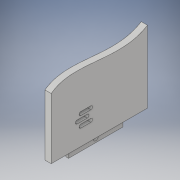
# Autodesk Inventor part: Case Left
Saved by Autodesk Inventor 2019 (Build 230136000, 136)
## iProperties
Created: 2022-04-25
Part Number: Case Left
Material: Generic
Document SubType Name: Modeling
Designer: Loxei
Density: 1 g/cm^3
Appearance: Default
Author: Loxei
Autodesk Inventor part; units mm, degrees
ref_plane "YZ Plane" through (0, 0, 0) normal (1, 0, 0) x (0, 1, 0)
ref_plane "XZ Plane" through (0, 0, 0) normal (0, 1, 0) x (-1, 0, 0)
ref_plane "XY Plane" through (0, 0, 0) normal (0, 0, 1) x (1, 0, 0)
sketch "Sketch2" plane through (0, 0, 0) normal (1, 0, 0) x (0, 1, 0)
  line L0 (43.74, 0) -> (-43.74, 0) construction
  line L1 (0, 65.172) -> (0, -65.172) construction
  spline S0 degree 3 poles (-5.8666, 35) (13.8832, 21.2522) (-10.0462, -16.0043) (8.551, -35) knots 1 1 1 1 2 2 2 2
  line L2 (-5.8666, 35) -> (13.8832, 21.2522) construction
  line L3 (13.8832, 21.2522) -> (-10.0462, -16.0043) construction
  line L4 (-10.0462, -16.0043) -> (8.551, -35) construction
  line L5 (-5.8666, 35) -> (-40.8666, 35)
  line L6 (-40.8666, 35) -> (-40.8666, 31)
  line L7 (-40.8666, 31) -> (-1.7165, 31)
  line L8 (-40.8666, 31) -> (-40.8666, -35)
  line L9 (-40.8666, -35) -> (8.551, -35)
  line L10 (-40.8666, -31) -> (5.392, -31)
  point P0 (0, 0)
  point P1 (0, 0)
  point P2 (0, 0)
  point P3 (0, 0)
  point P4 (-1.7165, 31)
  dimension "d0" = 35
  dimension "d1" = 4
  dimension "d2" = 4
  constraints: 16 end point, 4 midpoint, 3 perpendicular, 3 vertical, 2 horizontal, 2 parallel, 2 symmetric about line, 1 point on line, 6 other
  measures "d0" distance of L2.start L5.end
  measures "d1" distance of L5.end L6.end
  measures "d2" distance of L8.end L10.start
extrude "Extrusion1" add sketch "Sketch2" along normal blind 4 contours S0 L10 L8 L7
sketch "Sketch3" plane through (0, -40.8666, -31) normal (0, -1, 0) x (1, 0, 0)
  line L0 (0, 62) -> (0, 0) projected
  line L1 (0, 48.5) -> (1.7, 48.5)
  line L2 (1.7, 48.5) -> (1.7, 13.5)
  line L3 (1.7, 13.5) -> (0, 13.5)
  line L4 (0, 13.5) -> (0, 48.5)
  line L5 (0, 62) -> (4, 62) projected
  line L6 (0, 0) -> (4, 0) projected
  point P0 (0, 31)
  dimension "d5" = 1.7
  dimension "d6" = 35
  dimension "d7" = 13.5
  dimension "d8" = 13.5
  constraints: 8 end point, 2 parallel, 1 horizontal, 1 perpendicular, 1 point on line
  measures "d5" distance of L2.end L3.end
  measures "d6" distance of L1.end L2.end
  measures "d7" distance from line of L5 L1.start
  measures "d8" distance between parallel lines of L6 L3
extrude "Extrusion2" add sketch "Sketch3" along normal blind 4.9
chamfer "Chamfer1" distance 1.5 angle 45 1 edges at (1.7, -40.8666, 0)
sketch "Sketch4" plane through (0, 0, 0) normal (-1, 0, 0) x (0, 0, 1)
  circle A0 centre (22.15, -13.9166) radius 1.15
  circle A1 centre (22.15, -37.9166) radius 1.15
  line L0 (22.15, -13.9166) -> (22.15, -37.9166) construction
  circle A2 centre (-28.65, -13.9166) radius 1.15
  circle A3 centre (-28.65, -37.9166) radius 1.15
  line L1 (-28.65, -13.9166) -> (-28.65, -37.9166) construction
  line L2 (-28.65, -25.9166) -> (22.15, -25.9166) construction
  line L3 (-31, -40.8666) -> (-31, 5.392) projected
  line L4 (-17.5, -40.8666) -> (-31, -40.8666) projected
  point P0 (0, 0)
  dimension "d14" = 2.3
  dimension "d15" = 2.3
  dimension "d16" = 24
  dimension "d17" = 2.3
  dimension "d18" = 2.3
  dimension "d19" = 24
  dimension "d20" = 50.8
  dimension "d21" = 2.35
  dimension "d22" = 2.95
  constraints: 6 end point, 4 centre point, 2 midpoint, 2 vertical, 1 perpendicular
  measures "d14" diameter of A0
  measures "d15" diameter of A1
  measures "d16" distance of L0.start L0.end
  measures "d17" diameter of A2
  measures "d18" diameter of A3
  measures "d19" distance of L1.start L1.end
  measures "d20" distance of L2.start L2.end
  measures "d21" distance between parallel lines of L3 L1
  measures "d22" distance from line of L4 L1.end
extrude "Extrusion3" add sketch "Sketch4" along normal blind 8
sketch "Sketch6" plane through (0, 0, 0) normal (-1, 0, 0) x (0, 0, 1)
  line L0 (5.4658, -29.4166) -> (11.9658, -29.4166) construction
  line L1 (5.4658, -30.5146) -> (11.9658, -30.5146)
  line L2 (11.9658, -28.3186) -> (5.4658, -28.3186)
  arc A0 (5.4658, -28.3186) -> (5.4658, -30.5146) centre (5.4658, -29.4166) ccw
  arc A1 (11.9658, -30.5146) -> (11.9658, -28.3186) centre (11.9658, -29.4166) ccw
  line L3 (7.7658, -25.9166) -> (14.3248, -25.9166) construction
  line L4 (7.7658, -27.0146) -> (14.3248, -27.0146)
  line L5 (14.3248, -24.8186) -> (7.7658, -24.8186)
  arc A2 (7.7658, -24.8186) -> (7.7658, -27.0146) centre (7.7658, -25.9166) ccw
  arc A3 (14.3248, -27.0146) -> (14.3248, -24.8186) centre (14.3248, -25.9166) ccw
  line L6 (5.4658, -22.4166) -> (11.9658, -22.4166) construction
  line L7 (5.4658, -23.5146) -> (11.9658, -23.5146)
  line L8 (11.9658, -21.3186) -> (5.4658, -21.3186)
  arc A4 (5.4658, -21.3186) -> (5.4658, -23.5146) centre (5.4658, -22.4166) ccw
  arc A5 (11.9658, -23.5146) -> (11.9658, -21.3186) centre (11.9658, -22.4166) ccw
  line L9 (8.7158, -34.2999) -> (8.7158, -18.7387) construction
  circle A6 centre (22.15, -13.9166) radius 1.15 projected
  circle A7 centre (22.15, -37.9166) radius 1.15 projected
  point P0 (0, 0)
  point P1 (8.7158, -29.4166)
  point P2 (11.0453, -25.9166)
  point P3 (8.7158, -22.4166)
  dimension "d25" = 6.5
  dimension "d26" = 2.3
  dimension "d27" = 6.5
  dimension "d28" = 12
  dimension "d29" = 12
  dimension "d32" = 3.5
  constraints: 26 end point, 12 point on circle, 12 tangent, 6 centre point, 3 horizontal, 3 midpoint, 3 parallel, 2 point on line, 1 perpendicular, 1 other
  measures "d25" distance of L0.start L0.end
  measures "d26" horizontal distance of L0.start L3.start
  measures "d27" distance of L6.start L6.end
  measures "d28" distance from line of A6.centre L3
  measures "d29" distance from line of A7.centre L3
  measures "d32" vertical distance of point (8.716, -29.417) point (11.045, -25.917)
extrude "Extrusion4" cut sketch "Sketch6" against normal blind 4 contours A0 L2 A1 L1 | A2 L5 A3 L4 | A4 L8 A5 L7
sketch "Sketch7" plane through (0, 0, 0) normal (-1, 0, 0) x (0, 0, 1)
  line L0 (-17.5, -40.8666) -> (17.5, -40.8666) projected
  circle A0 centre (0, -43.1166) radius 1.575
  point P0 (0, 0)
  dimension "d33" = 2.25
  dimension "d34" = 3.15
  constraints: 1 centre point
  measures "d33" distance from line of L0 A0.centre
  measures "d34" diameter of A0
extrude "Extrusion5" cut sketch "Sketch7" against normal blind 4
fillet "Fillet2" radius 0.5 4 edges at (-8, -13.9166, -29.8) (-8, -13.9166, 21) (-8, -37.9166, 21) (-8, -37.9166, -29.8)
chamfer "Chamfer2" distance 2 angle 45 4 edges at (0, -37.9166, -29.8) (0, -13.9166, -29.8) (0, -13.9166, 21) (0, -37.9166, 21)
fillet "Fillet3" radius 2 4 edges at (-2, -37.9166, 21) (-2, -13.9166, 21) (-2, -13.9166, -29.8) (-2, -37.9166, -29.8)
equation "\"d7\" = d8"
equation "\"d27\" = d25"
equation "\"d28\" = d29"
body "Solid1"
